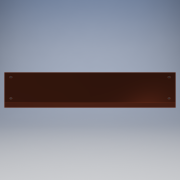
# Autodesk Inventor part: mount-base
Saved by Autodesk Inventor 2017 SP1 (Build 210196100, 196)
## iProperties
Created: 2017-02-03
Part Number: mount-base
Material: Copper
Document SubType Name: Modeling
Designer: Alex
Density: 8.94 g/cm^3
Appearance: Copper - Polished
Author: Alex
Autodesk Inventor part; units mm, degrees
ref_plane "YZ Plane" through (0, 0, 0) normal (1, 0, 0) x (0, 1, 0)
ref_plane "XZ Plane" through (0, 0, 0) normal (0, 1, 0) x (-1, 0, 0)
ref_plane "XY Plane" through (0, 0, 0) normal (0, 0, 1) x (1, 0, 0)
sketch "Sketch1" plane through (0, 0, 0) normal (0, 1, 0) x (-1, 0, 0)
  line L0 (10, 40) -> (-10, 40)
  line L1 (-10, 40) -> (-10, -40)
  line L2 (-10, -40) -> (10, -40)
  line L3 (10, -40) -> (10, 40)
  line L4 (10, 40) -> (-10, -40) construction
  line L5 (-10, 40) -> (10, -40) construction
  point P0 (0, 0)
  dimension "height" = 20
  dimension "width" = 80
  constraints: 12 end point, 2 midpoint, 2 parallel, 1 horizontal, 1 perpendicular
  measures "height" distance of L2.end L1.end
  measures "width" distance of L1.end L0.end
extrude "Extrusion1" add sketch "Sketch1" along normal blind 3
sketch "Sketch3" plane through (0, 3, 0) normal (0, 1, 0) x (1, 0, 0)
  line L0 (-7, -37) -> (7, -37) construction
  line L1 (7, -37) -> (7, 37) construction
  line L2 (7, 37) -> (-7, 37) construction
  line L3 (-7, 37) -> (-7, -37) construction
  line L4 (-7, -37) -> (7, 37) construction
  line L5 (7, -37) -> (-7, 37) construction
  line L6 (-10, -40) -> (10, -40) projected
  line L7 (-10, 40) -> (-10, -40) projected
  point P0 (0, 0)
  dimension "d4" = 3
  dimension "d5" = 3
  constraints: 12 end point, 2 midpoint, 2 parallel, 1 horizontal, 1 perpendicular
  measures "d4" distance between parallel lines of L6 L0
  measures "d5" distance between parallel lines of L7 L3
hole "Hole1" at (-7, 3, 37) at (7, 3, 37) at (7, 3, -37) at (-7, 3, -37) direction (0, -1, 0) diameter 1.567 end through all thread size "M2x0.4" class "6H" standard "ISO Metric profile"
body "Solid1"
